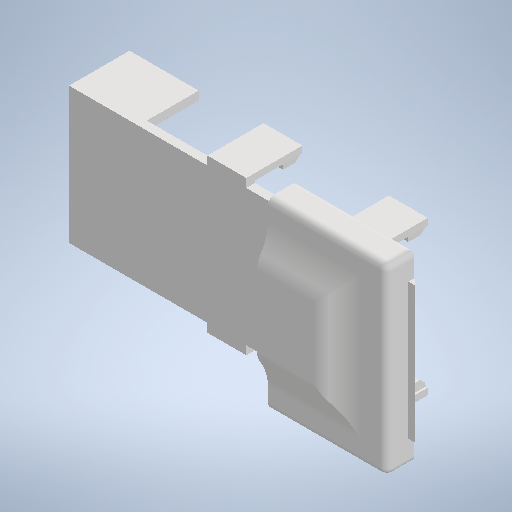
# Autodesk Inventor part: np2_cap_no_headstage_top
Saved by Autodesk Inventor 2025 (Build 290162000, 162)
## iProperties
Created: 2023-11-21
Part Number: np2_cap_no_headstage_top
Material: Generic
Document SubType Name: Modeling
Designer: mmelin
Density: 1 g/cm^3
Appearance: Default
Author: mmelin
Autodesk Inventor part; units mm, degrees
ref_plane "YZ Plane" through (0, 0, 0) normal (1, 0, 0) x (0, 1, 0)
ref_plane "XZ Plane" through (0, 0, 0) normal (0, 1, 0) x (-1, 0, 0)
sketch "Sketch1" plane through (0, 0, 0) normal (0, 0, 1) x (1, 0, 0)
  line L0 (1, -0.6319) -> (1, -5.5819) projected
  line L1 (-15, 0) -> (-11.6, 0)
  line L2 (-6.8, -6.3) -> (-8.6, -6.3) projected
  line L3 (-8.6, 0) -> (-6.8, 0) projected
  line L4 (-2.8, 0) -> (-1, 0) projected
  line L5 (-6.8, -6.3) -> (-8.6, -6.3) projected
  line L6 (-1, -6.3) -> (-2.8, -6.3) projected
  line L7 (-8.6, -6.3) -> (-6.8, -6.3)
  line L8 (-6.8, -6.3) -> (-6.8, -6.7)
  line L9 (-6.8, -6.7) -> (-8.6, -6.7)
  line L10 (-8.6, -6.7) -> (-8.6, -6.3)
  line L11 (-8.6, 0) -> (-6.8, 0)
  line L12 (-6.8, 0) -> (-6.8, 0.4)
  line L13 (-6.8, 0.4) -> (-8.6, 0.4)
  line L14 (-8.6, 0.4) -> (-8.6, 0)
  line L15 (-2.8, 0) -> (-1, 0)
  line L16 (-1, 0) -> (-1, 0.4)
  line L17 (-1, 0.4) -> (-2.8, 0.4)
  line L18 (-2.8, 0.4) -> (-2.8, 0)
  line L19 (-2.8, -6.3) -> (-1, -6.3)
  line L20 (-1, -6.3) -> (-1, -6.7)
  line L21 (-1, -6.7) -> (-2.8, -6.7)
  line L22 (-2.8, -6.7) -> (-2.8, -6.3)
  line L23 (-8.6, -5.9) -> (-8.6, -6.3) projected
  line L24 (-6.8, -5.9) -> (-6.8, -6.3) projected
  line L25 (-2.8, -5.9) -> (-2.8, -6.3) projected
  line L26 (-1, -5.9) -> (-1, -6.3) projected
  line L27 (1, -6.3) -> (-15, -6.3)
  line L28 (-15, -6.3) -> (-15, 0)
  line L29 (-15, 0) -> (1, 0)
  line L30 (1, 0) -> (1, -6.3)
  line L31 (-15, -1.7791) -> (-15, -4.5209) projected
  point P0 (0, 0)
  point P1 (1, -5.5819)
  point P2 (1, -0.6319)
  dimension "d2" = 0.4
  constraints: 42 end point, 16 collinear, 10 parallel, 5 horizontal, 5 perpendicular, 3 equal length
  measures "d2" distance of L7.end L8.end
extrude "Extrusion1" add sketch "Sketch1" along normal blind 0.4
sketch "Sketch2" plane through (0, 0, 0) normal (0, 0, -1) x (-1, 0, 0)
  line L0 (8.6, -6.7) -> (6.8, -6.7) projected
  line L1 (6.8, -6.7) -> (6.8, -6.3) projected
  line L2 (8.6, -6.7) -> (6.8, -6.7)
  line L3 (6.8, -6.7) -> (6.8, -6.4)
  line L4 (6.8, -6.4) -> (8.6, -6.4)
  line L5 (8.6, -6.4) -> (8.6, -6.7)
  line L6 (2.8, -6.3) -> (2.8, -6.7) projected
  line L7 (1, -6.7) -> (1, -6.3) projected
  line L8 (2.8, -6.7) -> (1, -6.7)
  line L9 (1, -6.7) -> (1, -6.4)
  line L10 (1, -6.4) -> (2.8, -6.4)
  line L11 (2.8, -6.4) -> (2.8, -6.7)
  line L12 (1, 0) -> (1, 0.4) projected
  line L13 (2.8, 0.4) -> (2.8, 0) projected
  line L14 (1, 0.4) -> (2.8, 0.4)
  line L15 (2.8, 0.4) -> (2.8, 0.1)
  line L16 (2.8, 0.1) -> (1, 0.1)
  line L17 (1, 0.1) -> (1, 0.4)
  line L18 (6.8, 0.4) -> (8.6, 0.4) projected
  line L19 (8.6, 0.4) -> (8.6, 0) projected
  line L20 (6.8, 0.4) -> (8.6, 0.4)
  line L21 (8.6, 0.4) -> (8.6, 0.1)
  line L22 (8.6, 0.1) -> (6.8, 0.1)
  line L23 (6.8, 0.1) -> (6.8, 0.4)
  line L24 (6.8, -6.3) -> (2.8, -6.3) projected
  line L25 (2.8, 0) -> (6.8, 0) projected
  point P0 (0, 0)
  dimension "d3" = 0.1
  dimension "d4" = 0.1
  constraints: 32 end point, 8 parallel, 4 horizontal, 4 perpendicular, 4 point on line, 2 collinear
  measures "d3" distance between parallel lines of L4 L24
  measures "d4" distance between parallel lines of L25 L22
ref_plane "Work Plane1" through (-8.6, -0.4, -2.2) normal (0, 0, 1) x (1, 0, 0)
extrude "Extrusion2" add sketch "Sketch2" along normal up to surface (2.2 mm away)
sketch "Sketch3" plane through (-8.6, 0.1, 0) normal (0, -1, 0) x (1, 0, 0)
  line L0 (0.1, -1.4) -> (1.7, -1.4)
  line L1 (1.7, -1.4) -> (1.7, -2.2)
  line L2 (1.7, -2.2) -> (0.1, -2.2)
  line L3 (0.1, -2.2) -> (0.1, -1.4)
  line L4 (5.9, -1.4) -> (7.5, -1.4)
  line L5 (7.5, -1.4) -> (7.5, -2.2)
  line L6 (7.5, -2.2) -> (5.9, -2.2)
  line L7 (5.9, -2.2) -> (5.9, -1.4)
  line L8 (1.8, -2.2) -> (1.8, -1.2) projected
  line L9 (1.8, -1.2) -> (0, -1.2) projected
  line L10 (0, -2.2) -> (1.8, -2.2) projected
  line L11 (0, -1.2) -> (0, -2.2) projected
  line L12 (7.6, -2.2) -> (7.6, -1.2) projected
  line L13 (5.8, -2.2) -> (7.6, -2.2) projected
  line L14 (7.6, -1.2) -> (5.8, -1.2) projected
  line L15 (5.8, -1.2) -> (5.8, -2.2) projected
  line L16 (1.8, -2.2) -> (0, -2.2) projected
  line L17 (7.6, -2.2) -> (5.8, -2.2) projected
  point P0 (8.6, 0)
  point P1 (6.7, -1.2)
  dimension "d7" = 0.1
  dimension "d8" = 0.2
  dimension "d9" = 0.1
  dimension "d10" = 0.1
  dimension "d11" = 0.2
  dimension "d12" = 0.1
  constraints: 16 end point, 4 parallel, 2 collinear, 2 horizontal, 2 perpendicular, 1 midpoint
  measures "d7" distance between parallel lines of L11 L3
  measures "d8" distance between parallel lines of L9 L0
  measures "d9" distance between parallel lines of L8 L1
  measures "d10" distance between parallel lines of L15 L7
  measures "d11" distance from line of point (6.7, -1.2) L4
  measures "d12" distance between parallel lines of L12 L5
extrude "Extrusion3" add sketch "Sketch3" along normal blind 0.35 draft -5 contours L0 L1 L2 L3 | L4 L5 L6 L7
sketch "Sketch4" plane through (-2.8, -6.4, 0) normal (0, 1, 0) x (1, 0, 0)
  line L0 (-4.1, 2.2) -> (-5.7, 2.2) projected
  line L1 (-5.7, 2.2) -> (-5.7, 1.4) projected
  line L2 (-4.1, 1.4) -> (-4.1, 2.2) projected
  line L3 (-5.7, 1.4) -> (-4.1, 1.4) projected
  line L4 (0.1, 1.4) -> (1.7, 1.4) projected
  line L5 (0.1, 2.2) -> (0.1, 1.4) projected
  line L6 (1.7, 2.2) -> (0.1, 2.2) projected
  line L7 (1.7, 1.4) -> (1.7, 2.2) projected
  point P0 (2.8, 0)
extrude "Extrusion4" add sketch "Sketch4" along normal blind 0.35 draft -5
chamfer "Chamfer1" distance 0.2 angle 45 4 edges at (-1.9, -0.25, -2.1694) (-7.7, -0.25, -2.1694) (-1.9, -6.05, -2.1694) (-7.7, -6.05, -2.1694)
sketch "Sketch5" plane through (0, 0, 0) normal (0, 0, -1) x (-1, 0, 0)
  line L0 (15, -6.3) -> (11.8, -6.3)
  line L1 (11.8, -6.3) -> (11.8, -5.9)
  line L2 (11.8, -5.9) -> (15, -5.9)
  line L3 (15, -5.9) -> (15, -6.3)
  line L4 (8.6, 0) -> (15, 0) projected
  line L5 (15, 0) -> (11.8, 0)
  line L6 (11.8, 0) -> (11.8, -0.4)
  line L7 (11.8, -0.4) -> (15, -0.4)
  line L8 (15, -0.4) -> (15, 0)
  line L9 (11.6, 0) -> (11.6, -0.4) projected
  line L10 (11.6, -5.9) -> (11.6, -6.3) projected
  point P0 (0, 0)
  dimension "d20" = 0.2
  dimension "d21" = 0.2
  constraints: 16 end point, 6 parallel, 2 horizontal, 2 perpendicular
  measures "d20" distance between parallel lines of L6 L9
  measures "d21" distance between parallel lines of L10 L1
extrude "Extrusion5" add sketch "Sketch5" along normal blind 2.4
sketch "Sketch6" plane through (0, 0, 0) normal (0, 0, -1) x (-1, 0, 0)
  line L0 (15, -0.4) -> (15, -5.9) projected
  line L1 (15, -5.9) -> (14.7, -5.9)
  line L2 (14.7, -5.9) -> (14.7, -0.4)
  line L3 (14.7, -0.4) -> (15, -0.4)
  line L4 (15, -0.4) -> (15, -5.9)
  line L5 (15, -0.4) -> (11.8, -0.4) projected
  point P0 (0, 0)
  dimension "d24" = 0.3
  constraints: 8 end point, 2 parallel, 1 collinear, 1 horizontal, 1 perpendicular
  measures "d24" distance between parallel lines of L4 L2
extrude "Extrusion6" add sketch "Sketch6" along normal blind 2.1
sketch "Sketch7" plane through (0, 0, 0.4) normal (0, 0, 1) x (1, 0, 0)
  line L0 (-4.8, 1.1) -> (0.7, 1.1)
  line L1 (0.7, 1.1) -> (0.7, -7.4)
  line L2 (0.7, -7.4) -> (-4.8, -7.4)
  line L3 (-4.8, -7.4) -> (-4.8, 1.1)
  line L4 (-14.7, -5.9) -> (-14.7, -0.4) projected
  line L5 (1, -6.3) -> (1, 0) projected
  point P0 (0, 0)
  point P1 (-14.7, -3.15)
  dimension "d27" = 8.5
  dimension "d28" = 4.25
  dimension "d29" = 5.5
  dimension "d30" = 0.3
  constraints: 8 end point, 2 parallel, 1 horizontal, 1 midpoint, 1 perpendicular
  measures "d27" distance of L0.end L1.end
  measures "d28" distance from line of L0 point (-14.7, -3.15)
  measures "d29" distance of L1.end L2.end
  measures "d30" distance between parallel lines of L1 L5
extrude "Extrusion7" add sketch "Sketch7" along normal blind 1 and the other way blind 0.4
sketch "Sketch8" plane through (-4.8, -6.3, 0.4) normal (-1, 0, 0) x (0, 0, 1)
  line L0 (0.7, 7.1) -> (-0.1, 7.1)
  line L1 (-0.1, 7.1) -> (-0.1, -0.8)
  line L2 (-0.1, -0.8) -> (0.7, -0.8)
  line L3 (0.7, -0.8) -> (0.7, 7.1)
  line L4 (1, 7.4) -> (1, -1.1) projected
  line L5 (-0.4, 6.3) -> (-0.4, 7.4) projected
  line L6 (1, 7.4) -> (-0.4, 7.4) projected
  line L7 (-0.4, -1.1) -> (1, -1.1) projected
  point P0 (-0.4, 6.85)
  point P1 (0.3, 7.1)
  point P2 (0.3, 7.4)
  point P3 (0.3, -1.1)
  point P4 (0.3, -0.8)
  dimension "d35" = 0.3
  dimension "d36" = 0.3
  dimension "d37" = 0.3
  dimension "d38" = 0.3
  constraints: 8 end point, 5 midpoint, 2 parallel, 1 horizontal, 1 perpendicular
  measures "d35" distance between parallel lines of L4 L3
  measures "d36" distance from line of point (-0.4, 6.85) L1
  measures "d37" distance of point (0.3, 7.1) point (0.3, 7.4)
  measures "d38" distance of point (0.3, -1.1) point (0.3, -0.8)
extrude "Extrusion8" cut sketch "Sketch8" against normal blind 5.1
fillet "Fillet1" radius 0.2 3 edges at (-2.25, 0.8, 1.1) (-2.25, -7.1, 1.1) (-2.25, -7.1, 0.3)
fillet "Fillet2" radius 0.3 7 edges at (-2.05, -7.4, 1.4) (-2.05, 1.1, 1.4) (-2.05, 1.1, 0) (-2.05, -7.4, 0) (0.7, -7.4, 0.7) (0.7, -3.15, 1.4) (0.7, 1.1, 0.7)
sketch "Sketch9" plane through (0, 0, 0) normal (0, 0, -1) x (-1, 0, 0)
  point P0 (0, 0)
sketch "Sketch10" plane through (0, 0, 0) normal (0, 0, -1) x (-1, 0, 0)
  line L0 (3.9, -0.65) -> (0.0657, -0.65)
  line L1 (0.0657, -0.65) -> (0.0657, -5.65)
  line L2 (0.0657, -5.65) -> (3.9, -5.65)
  line L3 (3.9, -5.65) -> (3.9, -0.65)
  line L4 (4.5, 0.5) -> (4.5, -6.8) projected
  line L5 (2.6694, -0.25) -> (1.1306, -0.25) projected
  line L6 (2.6694, -6.05) -> (1.1306, -6.05) projected
  line L7 (-0.7, 0.8) -> (-0.7, 0) projected
  point P0 (-1, 0.8)
  point P1 (-1, -7.1)
  dimension "d49" = 0.6
  dimension "d51" = 0.4
  dimension "d53" = 0.4
  dimension "d54" = 0.7658
  constraints: 8 end point, 2 parallel, 1 horizontal, 1 perpendicular, 1 other
  measures "d49" distance between parallel lines of L4 L3
  measures "d51" distance between parallel lines of L5 L0
  measures "d53" distance between parallel lines of L6 L2
extrude "Extrusion9" cut sketch "Sketch10" against normal up to surface (0.4 mm away)
fillet "Fillet4" radius 1 4 edges at (-3.9, -0.65, 0.15) (-0.0657, -0.65, 0.15) (-0.0657, -5.65, 0.15) (-3.9, -5.65, 0.15)
fillet "Fillet5" radius 1 1 edges at (1, -3.15, 0)
sketch "Sketch11" plane through (-4.8, 0, 0) normal (-1, 0, 0) x (0, 0, 1)
  arc A0 (1.1, -7.4) -> (1.4, -7.1) centre (1.1, -7.1) ccw projected
  line L0 (1.4, 0.8) -> (1.4, -7.1) projected
  arc A1 (1.4, 0.8) -> (1.1, 1.1) centre (1.1, 0.8) ccw projected
  line L1 (1.1, 1.1) -> (0.3, 1.1) projected
  arc A2 (0.3, 1.1) -> (0, 0.8) centre (0.3, 0.8) ccw projected
  line L2 (0, 0) -> (0, 0.8) projected
  line L3 (0.3, 0) -> (0, 0) projected
  line L4 (0.3, 0.8) -> (0.9, 0.8) projected
  arc A3 (1.1, 0.6) -> (0.9, 0.8) centre (0.9, 0.6) ccw projected
  line L5 (1.1, 0.6) -> (1.1, -6.9) projected
  arc A4 (0.9, -7.1) -> (1.1, -6.9) centre (0.9, -6.9) ccw projected
  line L6 (0.9, -7.1) -> (0.5, -7.1) projected
  arc A5 (0.3, -6.9) -> (0.5, -7.1) centre (0.5, -6.9) ccw projected
  line L7 (0, -6.3) -> (0.3, -6.3) projected
  line L8 (0, -7.1) -> (0, -6.3) projected
  arc A6 (0, -7.1) -> (0.3, -7.4) centre (0.3, -7.1) ccw projected
  line L9 (0.3, -7.4) -> (1.1, -7.4) projected
  line L10 (1.9, -5.65) -> (1.4, -5.65)
  line L11 (1.4, -5.65) -> (1.4, -0.65)
  line L12 (1.4, -0.65) -> (1.9, -0.65)
  line L13 (1.9, -0.65) -> (1.9, -5.65)
  line L14 (0.3, 0) -> (0.3, 0.8) projected
  line L15 (0.3, -6.9) -> (0.3, -6.3) projected
  point P0 (1.1, -3.15)
  point P1 (1.9, -3.15)
  point P2 (1.4, -0.65)
  dimension "d61" = 0.5
  dimension "d62" = 0
  dimension "d63" = 5
  dimension "d64" = 0
  constraints: 8 end point, 2 midpoint, 2 parallel, 1 horizontal, 1 perpendicular
  measures "d61" distance of L11.end L12.end
  measures "d62" distance between parallel lines of L0 L11
  measures "d63" distance of L12.end L10.start
  measures "d64" vertical distance of point (1.1, -3.15) point (1.9, -3.15)
extrude "Extrusion10" add sketch "Sketch11" against normal blind 3.5 contours L0 L12 L13 L10
fillet "Fillet6" radius 1 3 edges at (-3.05, -0.65, 1.9) (-1.3, -3.15, 1.9) (-3.05, -5.65, 1.9)
sketch "Sketch12" plane through (-4.8, 0, 0) normal (-1, 0, 0) x (0, 0, 1)
  circle A0 centre (-3.9288, -3.05) radius 5.5288
  line L0 (1.1, 0.6) -> (1.1, -6.9) projected
  line L1 (1.1, -5.3476) -> (1.1, -0.7524)
  point P0 (0, 0)
  constraints: 2 end point, 2 point on circle, 2 point on line, 1 centre point
extrude "Extrusion11" cut sketch "Sketch12" against normal blind 3 contours A0 L0 picked at (1.192, -3.5694)
fillet "Fillet7" radius 2 3 edges at (-3.05, -0.65, 1.4) (-1.3, -3.15, 1.4) (-3.05, -5.65, 1.4)
fillet "Fillet8" radius 2 3 edges at (-3.3, -0.7524, 1.1) (-3.3, -5.3476, 1.1) (-1.8, -3.05, 1.6)
equation "\"d8\" = d11"
equation "\"d9\" = d7"
equation "\"d10\" = d7"
equation "\"d12\" = d7"
equation "\"d21\" = d20"
equation "\"d28\" = 0.5 * d27"
equation "\"d36\" = d35"
equation "\"d37\" = d35"
equation "\"d38\" = d37"
body "Solid1"
